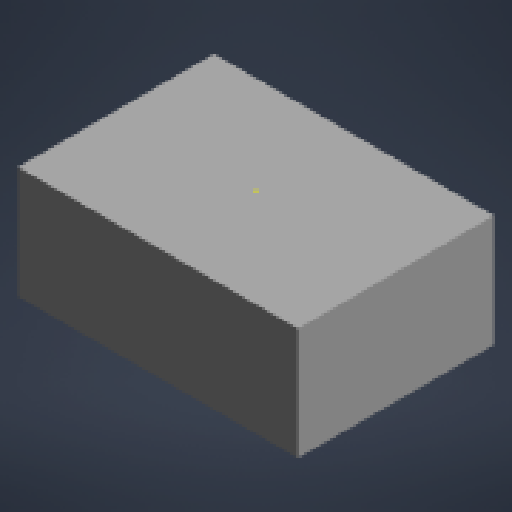
# Autodesk Inventor part: SpinCoater
Saved by Autodesk Inventor 2024.2 (Build 282272000, 272)
## iProperties
Created: 2024-10-04
Part Number: SpinCoater
Material: Generic
Document SubType Name: Modeling
Designer: jerem
Density: 1 g/cm^3
Appearance: Default
Author: jerem
Autodesk Inventor part; units mm, degrees
ref_plane "YZ Plane" through (0, 0, 0) normal (1, 0, 0) x (0, 1, 0)
ref_plane "XZ Plane" through (0, 0, 0) normal (0, 1, 0) x (-1, 0, 0)
ref_plane "XY Plane" through (0, 0, 0) normal (0, 0, 1) x (1, 0, 0)
sketch "Sketch1" plane through (0, 0, 0) normal (0, 1, 0) x (-1, 0, 0)
  line L0 (-125, -87.5) -> (125, -87.5)
  line L1 (125, -87.5) -> (125, 87.5)
  line L2 (125, 87.5) -> (-125, 87.5)
  line L3 (-125, 87.5) -> (-125, -87.5)
  line L4 (-125, -87.5) -> (125, 87.5) construction
  line L5 (125, -87.5) -> (-125, 87.5) construction
  point P0 (0, 0)
  dimension "d0" = 175
  dimension "d1" = 250
  constraints: 12 end point, 2 midpoint, 2 parallel, 1 horizontal, 1 perpendicular
  measures "d0" distance of L0.end L1.end
  measures "d1" distance of L1.end L2.end
extrude "Extrusion1" add sketch "Sketch1" along normal blind 100
sketch "Sketch2" plane through (0, 100, 0) normal (0, 1, 0) x (1, 0, 0)
  point P0 (0, 0)
sketch "Sketch3" plane through (0, 100, 0) normal (0, 1, 0) x (1, 0, 0)
  line L0 (-56.7304, 52.8714) -> (-40.2636, 52.8714) construction
  line L1 (-40.2636, 52.8714) -> (-40.2636, 42.5148) construction
  line L2 (-40.2636, 42.5148) -> (-56.7304, 42.5148) construction
  line L3 (-56.7304, 42.5148) -> (-56.7304, 52.8714) construction
  spline S0 degree 2 poles (-37.7272, 1.0886) (-43.1567, 1.0886) (-50.7742, 3.3576) (-54.1372, 4.9784) knots 0 0 0 1 2 2 2
  line L4 (-54.1372, 4.9784) -> (-54.1372, 13.3252)
  line L5 (-54.1372, 13.3252) -> (-53.651, 13.3252)
  spline S1 degree 2 poles (-53.651, 13.3252) (-50.369, 10.2458) (-42.0627, 6.8422) (-38.2134, 6.8422) knots 0 0 0 1 2 2 2
  spline S2 degree 2 poles (-38.2134, 6.8422) (-32.7028, 6.8422) (-27.0708, 11.4208) (-27.0708, 15.1891) knots 0 0 0 1 2 2 2
  spline S3 degree 2 poles (-27.0708, 15.1891) (-27.0708, 18.1874) (-30.0286, 21.9152) (-33.2296, 22.8471) knots 0 0 0 1 2 2 2
  spline S4 degree 2 poles (-33.2296, 22.8471) (-35.5392, 23.4954) (-39.3884, 24.3868) (-42.2652, 25.1161) knots 0 0 0 1 2 2 2
  spline S5 degree 2 poles (-42.2652, 25.1161) (-44.8584, 25.805) (-48.9508, 27.8714) (-50.5311, 29.5327) knots 0 0 0 1 2 2 2
  spline S6 degree 2 poles (-50.5311, 29.5327) (-52.0708, 31.1939) (-53.7725, 35.651) (-53.7725, 38.5683) knots 0 0 0 1 2 2 2
  spline S7 degree 2 poles (-53.7725, 38.5683) (-53.7725, 44.6461) (-44.2912, 52.8714) (-36.9573, 52.8714) knots 0 0 0 1 2 2 2
  spline S8 degree 2 poles (-36.9573, 52.8714) (-32.7434, 52.8714) (-25.2879, 51.2101) (-22.087, 49.6299) knots 0 0 0 1 2 2 2
  line L6 (-22.087, 49.6299) -> (-22.087, 41.6883)
  line L7 (-22.087, 41.6883) -> (-22.5732, 41.6883)
  spline S9 degree 2 poles (-22.5732, 41.6883) (-24.9638, 43.8763) (-32.4192, 47.1178) (-36.5116, 47.1178) knots 0 0 0 1 2 2 2
  spline S10 degree 2 poles (-36.5116, 47.1178) (-41.1307, 47.1178) (-46.8439, 42.7823) (-46.8439, 39.2571) knots 0 0 0 1 2 2 2
  spline S11 degree 2 poles (-46.8439, 39.2571) (-46.8439, 36.0967) (-43.4808, 32.3285) (-40.3204, 31.4776) knots 0 0 0 1 2 2 2
  spline S12 degree 2 poles (-40.3204, 31.4776) (-38.2134, 30.9103) (-32.0951, 29.4516) (-30.0691, 28.8439) knots 0 0 0 1 2 2 2
  spline S13 degree 2 poles (-30.0691, 28.8439) (-24.9233, 27.2636) (-20.1421, 20.9022) (-20.1421, 16.2426) knots 0 0 0 1 2 2 2
  spline S14 degree 2 poles (-20.1421, 16.2426) (-20.1421, 13.2847) (-22.5327, 7.6121) (-24.6802, 5.6267) knots 0 0 0 1 2 2 2
  spline S15 degree 2 poles (-24.6802, 5.6267) (-27.0708, 3.4387) (-33.1486, 1.0886) (-37.7272, 1.0886) knots 0 0 0 1 2 2 2
  spline S16 degree 2 poles (6.1545, 1.0886) (1.2923, 1.0886) (-6.933, 4.3706) (-9.9314, 7.6526) knots 0 0 0 1 2 2 2
  spline S17 degree 2 poles (-9.9314, 7.6526) (-12.9298, 10.8941) (-16.2118, 20.6186) (-16.2118, 26.9395) knots 0 0 0 1 2 2 2
  spline S18 degree 2 poles (-16.2118, 26.9395) (-16.2118, 33.2199) (-13.0108, 42.5392) (-9.9719, 45.9832) knots 0 0 0 1 2 2 2
  spline S19 degree 2 poles (-9.9719, 45.9832) (-6.9735, 49.3463) (1.2113, 52.8714) (6.2761, 52.8714) knots 0 0 0 1 2 2 2
  spline S20 degree 2 poles (6.2761, 52.8714) (8.7882, 52.8714) (13.2048, 52.1421) (15.0686, 51.5748) knots 0 0 0 1 2 2 2
  spline S21 degree 2 poles (15.0686, 51.5748) (16.6894, 51.0481) (20.0524, 49.5489) (21.7137, 48.6575) knots 0 0 0 1 2 2 2
  line L8 (21.7137, 48.6575) -> (21.7137, 40.6348)
  line L9 (21.7137, 40.6348) -> (21.1869, 40.6348)
  spline S22 degree 2 poles (21.1869, 40.6348) (20.2955, 41.4451) (17.5403, 43.7142) (15.5548, 44.8082) knots 0 0 0 1 2 2 2
  spline S23 degree 2 poles (15.5548, 44.8082) (13.6505, 45.8617) (9.1529, 47.1988) (6.2356, 47.1988) knots 0 0 0 1 2 2 2
  spline S24 degree 2 poles (6.2356, 47.1988) (3.0346, 47.1988) (-2.6785, 44.5651) (-4.826, 42.0529) knots 0 0 0 1 2 2 2
  spline S25 degree 2 poles (-4.826, 42.0529) (-6.933, 39.5003) (-9.2831, 31.7612) (-9.2831, 26.9395) knots 0 0 0 1 2 2 2
  spline S26 degree 2 poles (-9.2831, 26.9395) (-9.2831, 21.7936) (-6.8114, 14.3787) (-4.664, 11.826) knots 0 0 0 1 2 2 2
  spline S27 degree 2 poles (-4.664, 11.826) (-2.557, 9.3544) (3.0751, 6.8422) (6.2356, 6.8422) knots 0 0 0 1 2 2 2
  spline S28 degree 2 poles (6.2356, 6.8422) (9.1124, 6.8422) (14.0151, 8.2604) (15.9195, 9.3139) knots 0 0 0 1 2 2 2
  spline S29 degree 2 poles (15.9195, 9.3139) (17.7429, 10.3674) (20.4576, 12.5554) (21.2275, 13.3252) knots 0 0 0 1 2 2 2
  line L10 (21.2275, 13.3252) -> (21.7137, 13.3252)
  line L11 (21.7137, 13.3252) -> (21.7137, 5.3836)
  spline S30 degree 2 poles (21.7137, 5.3836) (20.0524, 4.6137) (17.1351, 3.1956) (15.0686, 2.5473) knots 0 0 0 1 2 2 2
  spline S31 degree 2 poles (15.0686, 2.5473) (12.8806, 1.8179) (9.1529, 1.0886) (6.1545, 1.0886) knots 0 0 0 1 2 2 2
  point P0 (0, 0)
  constraints: 1 coincident, 2 other
extrude "Extrusion2" cut sketch "Sketch3" against normal blind 10
body "Solid1"
